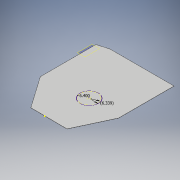
# Autodesk Inventor part: side cover plate Base
Saved by Autodesk Inventor 2018 (Build 220112000, 112)
## iProperties
Created: 2018-05-29
Part Number: side cover plate Base
Material: Generic
Document SubType Name: Modeling
Designer: p446024
Density: 1 g/cm^3
Appearance: Default
Author: p446024
Autodesk Inventor part; units mm, degrees
ref_plane "YZ Plane" through (0, 0, 0) normal (1, 0, 0) x (0, 1, 0)
ref_plane "XZ Plane" through (0, 0, 0) normal (0, 1, 0) x (-1, 0, 0)
ref_plane "XY Plane" through (0, 0, 0) normal (0, 0, 1) x (1, 0, 0)
ref_plane "Work Plane1" through (-244.5168, 0, -292.1078) normal (0, -1, 0) x (1, 0, 0)
sketch "Sketch1" plane through (-244.5168, 0, -292.1078) normal (0, -1, 0) x (1, 0, 0)
  line L0 (-82.2349, -443.0164) -> (-82.2349, 4.1434)
  line L1 (16.0565, -523.4999) -> (-89.6349, -493.4083) projected
  line L2 (-82.2349, 4.1434) -> (116.5991, 288.1078)
  line L3 (116.5991, 288.1078) -> (240.5168, 288.1078)
  line L4 (590.8332, -25.4546) -> (443.4975, 290.5078) projected
  line L5 (590.8332, -523.4999) -> (590.8332, -25.4546) projected
  point P0 (244.5168, 292.1078)
  constraints: 7 coincident, 6 end point
sketch "Sketch2" plane through (-244.5168, 0, -292.1078) normal (0, -1, 0) x (1, 0, 0)
  line L0 (16.0565, -523.4999) -> (-82.2349, -495.4665)
  line L1 (-82.2349, -495.4665) -> (-82.2349, 4.1434)
  line L2 (-82.2349, 4.1434) -> (116.5991, 288.1078)
  line L3 (116.5991, 288.1078) -> (443.4975, 290.5078)
  line L4 (443.4975, 290.5078) -> (590.8332, -25.4546)
  line L5 (590.8332, -25.4546) -> (590.8332, -523.4999)
  line L6 (590.8332, -523.4999) -> (16.0565, -523.4999)
  point P0 (244.5168, 292.1078)
  constraints: 14 end point, 1 parallel, 1 perpendicular, 1 vertical
extrude "Plate extrude" add sketch "Sketch2" against normal blind 1.6
sketch "Sketch3" plane through (-244.5168, 0, -292.1078) normal (0, -1, 0) x (1, 0, 0)
  circle A0 centre (303.4237, -47.9675) radius 80.5 construction
  circle A1 centre (303.4237, -47.7578) radius 75 construction
  line L0 (153.4237, 102.2422) -> (453.4237, 102.2422)
  line L1 (453.4237, 102.2422) -> (453.4237, -197.7578)
  line L2 (453.4237, -197.7578) -> (153.4237, -197.7578)
  line L3 (153.4237, -197.7578) -> (153.4237, 102.2422)
  line L4 (153.4237, 102.2422) -> (453.4237, -197.7578) construction
  line L5 (453.4237, 102.2422) -> (153.4237, -197.7578) construction
  point P0 (244.5168, 292.1078)
  dimension "d3" = 300
  dimension "d4" = 300
  constraints: 12 end point, 2 midpoint, 2 parallel, 1 horizontal, 1 perpendicular
  measures "d3" distance of L1.end L2.end
  measures "d4" distance of L0.end L1.end
extrude "Tailstock door" [suppressed]
sketch "Sketch4" plane through (-244.5168, 0, -292.1078) normal (0, -1, 0) x (1, 0, 0)
  circle A0 centre (303.4237, -47.7578) radius 75 construction
  circle A1 centre (303.4237, -47.7578) radius 81.28
  circle A2 centre (303.4237, -47.9675) radius 80.5 construction
  point P0 (244.5168, 292.1078)
  dimension "d7" = 162.56
  dimension "d8" = 161
  constraints: 1 centre point, 1 coincident
  measures "d7" diameter of A1
  measures "d8" diameter of A2
extrude "Headstock cut out" [suppressed]
sketch "Sketch5" plane through (-244.5168, 1.6, -292.1078) normal (0, 1, 0) x (1, 0, 0)
  point P0 (244.5168, -292.1078)
  point P1 (303.4237, 47.9675)
body "Solid1"
